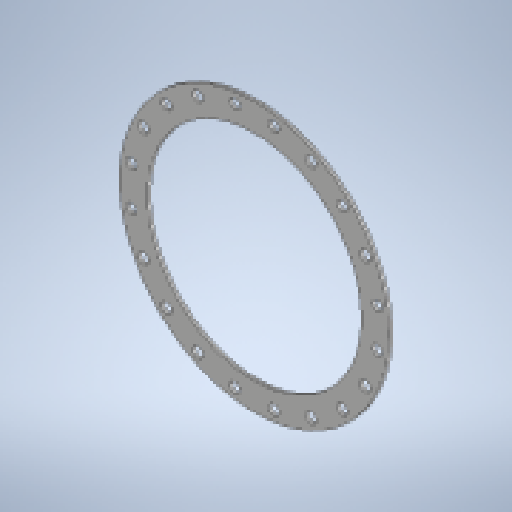
# Autodesk Inventor part: !!PRS 9512 accses hatch flangeipt_D1200
Saved by Autodesk Inventor 2026.2 (Build 302298000, 298)
## iProperties
Created: 2025-02-12
Part Number: !!PRS 9512 accses hatch flangeipt_D1200
Material: Generic
Document SubType Name: Sheet Metal
Designer: admin
Density: 1 g/cm^3
Flat Pattern Width: 67 cm
Flat Pattern Length: 67 cm
Flat Pattern Area: 4489 cm^2
Sheet Metal Rule: Default_mm
Sheet Metal Width: 670.000 mm
Sheet Metal Length: 670.000 mm
Sheet Metal Area: 448900.000 mm^2
Appearance: Default
Mass: 1023.51 g
Surface Area: 2989.04 cm^2
Volume: 1023.51 cm^3
Author: pokla
Autodesk Inventor part; units mm, degrees
ref_plane "YZ Plane" through (0, 0, 0) normal (1, 0, 0) x (0, 1, 0)
ref_plane "XZ Plane" through (0, 0, 0) normal (0, 1, 0) x (-1, 0, 0)
ref_plane "XY Plane" through (0, 0, 0) normal (0, 0, 1) x (1, 0, 0)
sketch "Sketch1" plane through (0, 0, 0) normal (0, 1, 0) x (-1, 0, 0)
  circle A0 centre (0, 0) radius 267
  circle A1 centre (0, 0) radius 335
  line L0 (335, 0) -> (267, 0)
  line L1 (-267, 0) -> (-335, 0)
  line L2 (0, 267) -> (0, 335)
  point P0 (301, 0)
  point P1 (-301, 0)
  point P2 (0, 301)
  dimension "d1" = 670
  dimension "d4" = 534
  constraints: 6 end point, 6 point on circle, 3 midpoint, 2 centre point, 2 coincident, 2 horizontal, 2 horizontal alignment, 1 vertical, 1 vertical alignment
  measures "d1" diameter of A1
  measures "d4" diameter of A0
extrude "Extrusion1" add sketch "Sketch1" along normal blind 8 contours L0 A1 L1 A0 | A0 L2 A1 L0 | A0 L1 A1 L2
sketch "Sketch2" plane through (0, 0, 0) normal (0, -1, 0) x (1, 0, 0)
  line L0 (0, 0) -> (0, 310) construction
  line L1 (0, 0) -> (48.4947, 306.1834) construction
  circle A0 centre (0, 0) radius 310 construction
  dimension "d14" = 620
  dimension "d15" = 9
  constraints: 4 end point, 2 coincident, 2 point on circle, 1 centre point, 1 vertical
  measures "d14" diameter of A0
  measures "d15" angle of L0 L1
hole "Hole1" at (48.4947, 0, 306.1834) direction (0, 1, 0) diameter 26 end through all
pattern_circular "Circular Pattern2" count 20 over 360 about axis through (0, -10, 0) along (0, 1, 0) of "Hole1"
equation "\"d2\" = Thickness"
equation "\"d21\" = Thickness"
equation "\"BendRadius\" = Thickness"
equation "\"BendReliefWidth\" = Thickness"
equation "\"BendReliefDepth\" = 0.5 * Thickness"
equation "\"CornerReliefSize\" = 4 * Thickness"
equation "\"MinimumRemnant\" = 2 * Thickness"
equation "\"TransitionRadius\" = BendRadius"
equation "\"JacobiRadiusSize\" = BendRadius"
equation "\"GapSize\" = Thickness"
equation "\"d8\" = Thickness"
equation "\"Thickness\" = 8"
body "Solid1"
